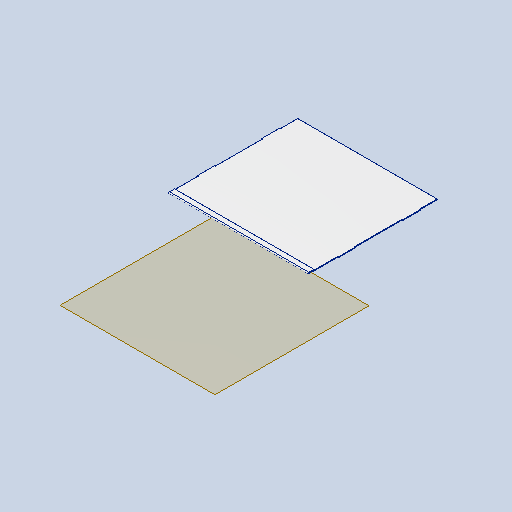
# Autodesk Inventor part: SHELVES
Saved by Autodesk Inventor 2025.2 (Build 292293000, 293)
## iProperties
Created: 2025-03-20
Part Number: SHELVES
Material: Aluminum 6061
Document SubType Name: Sheet Metal
Designer: bless
Density: 2.7 g/cm^3
Sheet Metal Rule: aluminum
Appearance: Aluminum - Flat
Flat Pattern Width: 58.2253 cm
Flat Pattern Length: 60.96 cm
Flat Pattern Area: 3549.42 cm^2
Sheet Metal Width: 22.923 in
Sheet Metal Length: 24.000 in
Sheet Metal Area: 550.161 in^2
Author: bless
Autodesk Inventor part; units mm, degrees
ref_plane "YZ Plane" through (0, 0, 0) normal (1, 0, 0) x (0, 1, 0)
ref_plane "XZ Plane" through (0, 0, 0) normal (0, 1, 0) x (-1, 0, 0)
ref_plane "XY Plane" through (0, 0, 0) normal (0, 0, 1) x (1, 0, 0)
ref_plane "Work Plane1" through (505.636, 20227.0512, -193.0762) normal (0, 1, 0) x (-1, 0, 0)
sketch "Sketch1" plane through (505.636, 20227.0512, -193.0762) normal (0, 1, 0) x (-1, 0, 0)
  circle A0 centre (-63.163, -692.5512) radius 4.7625
  circle A1 centre (-63.163, -444.9012) radius 4.7625
  circle A2 centre (-63.163, -321.0762) radius 4.7625
  circle A3 centre (-63.163, -568.7262) radius 4.7625
  circle A4 centre (-63.163, -816.3762) radius 4.7625
  circle A5 centre (495.637, -321.0762) radius 4.7625
  circle A6 centre (495.637, -444.9012) radius 4.7625
  circle A7 centre (495.637, -568.7262) radius 4.7625
  circle A8 centre (495.637, -692.5512) radius 4.7625
  circle A9 centre (495.637, -816.3762) radius 4.7625
  line L0 (443.2368, -260.7639) -> (-10.7628, -260.7639)
  line L1 (-10.7628, -260.7639) -> (-10.7628, -284.5637)
  line L2 (-10.7628, -284.5637) -> (-17.1128, -284.5637)
  line L3 (-17.1128, -284.5637) -> (-17.1128, -282.9762)
  line L4 (-88.563, -282.9762) -> (-17.1128, -282.9762)
  line L5 (-88.563, -867.1762) -> (-88.563, -282.9762)
  line L6 (521.037, -867.1762) -> (-88.563, -867.1762)
  line L7 (521.037, -282.9762) -> (521.037, -867.1762)
  line L8 (449.5868, -282.9762) -> (521.037, -282.9762)
  line L9 (449.5868, -282.9762) -> (449.5868, -284.5637)
  line L10 (449.5868, -284.5637) -> (443.2368, -284.5637)
  line L11 (443.2368, -284.5637) -> (443.2368, -260.7639)
  line L12 (521.037, -867.1762) -> (-88.563, -867.1762)
  line L13 (-88.563, -867.1762) -> (-88.563, -308.3762)
  line L14 (-88.563, -308.3762) -> (521.037, -308.3762)
  line L15 (521.037, -308.3762) -> (521.037, -867.1762)
  line L16 (-88.563, -790.9762) -> (-85.388, -790.9762)
  line L17 (-85.388, -790.9762) -> (-85.388, -714.7762)
  line L18 (-85.388, -714.7762) -> (-88.563, -714.7762)
  line L19 (-88.563, -714.7762) -> (-88.563, -790.9762)
  line L20 (-85.388, -511.5762) -> (-88.563, -511.5762)
  line L21 (-88.563, -511.5762) -> (-88.563, -435.3762)
  line L22 (-88.563, -435.3762) -> (-85.388, -435.3762)
  line L23 (-85.388, -435.3762) -> (-85.388, -511.5762)
  line L24 (-88.563, -308.3762) -> (-85.388, -308.3762)
  line L25 (-85.388, -308.3762) -> (-85.388, -435.3762)
  line L26 (-85.388, -435.3762) -> (-88.563, -435.3762)
  line L27 (-88.563, -435.3762) -> (-88.563, -308.3762)
  line L28 (-88.563, -511.5762) -> (-85.388, -511.5762)
  line L29 (-85.388, -511.5762) -> (-85.388, -714.7762)
  line L30 (-85.388, -714.7762) -> (-88.563, -714.7762)
  line L31 (-88.563, -714.7762) -> (-88.563, -511.5762)
  line L32 (521.037, -790.9762) -> (517.862, -790.9762)
  line L33 (517.862, -790.9762) -> (517.862, -714.7762)
  line L34 (517.862, -714.7762) -> (521.037, -714.7762)
  line L35 (521.037, -714.7762) -> (521.037, -790.9762)
  line L36 (521.037, -511.5762) -> (517.862, -511.5762)
  line L37 (517.862, -511.5762) -> (517.862, -435.3762)
  line L38 (517.862, -435.3762) -> (521.037, -435.3762)
  line L39 (521.037, -435.3762) -> (521.037, -511.5762)
  line L40 (521.037, -867.1762) -> (517.862, -867.1762)
  line L41 (517.862, -867.1762) -> (517.862, -790.9762)
  line L42 (517.862, -790.9762) -> (521.037, -790.9762)
  line L43 (521.037, -790.9762) -> (521.037, -867.1762)
  line L44 (521.037, -714.7762) -> (517.862, -714.7762)
  line L45 (517.862, -714.7762) -> (517.862, -511.5762)
  line L46 (517.862, -511.5762) -> (521.037, -511.5762)
  line L47 (521.037, -511.5762) -> (521.037, -714.7762)
  line L48 (521.037, -435.3762) -> (517.862, -435.3762)
  line L49 (517.862, -435.3762) -> (517.862, -308.3762)
  line L50 (517.862, -308.3762) -> (521.037, -308.3762)
  line L51 (521.037, -308.3762) -> (521.037, -435.3762)
  line L52 (-88.563, -790.9762) -> (-85.388, -790.9762)
  line L53 (-85.388, -790.9762) -> (-85.388, -867.1762)
  line L54 (-85.388, -867.1762) -> (-88.563, -867.1762)
  line L55 (-88.563, -867.1762) -> (-88.563, -790.9762)
  point P0 (505.636, 193.0762)
  point P1 (521.037, -714.7762)
  point P2 (521.037, -511.5762)
  point P3 (521.037, -435.3762)
  point P4 (-88.563, -435.3762)
  point P5 (-88.563, -511.5762)
  point P6 (-88.563, -714.7762)
  point P7 (-88.563, -790.9762)
  dimension "d0" = 609.6
  dimension "d1" = 558.8
  dimension "d2" = 76.2
  dimension "d3" = 76.2
  dimension "d4" = 3.175
  dimension "d5" = 355.6
  dimension "d6" = 76.2
  dimension "d7" = 3.175
  dimension "d8" = 3.175
  dimension "d9" = 76.2
  dimension "d10" = 76.2
  dimension "d11" = 3.175
  dimension "d12" = 76.2
  dimension "d13" = 355.6
  dimension "d14" = 3.175
  measures "d0" distance of L13.end L14.end
  measures "d1" distance of L12.end L13.end
  measures "d2" distance of L16.end L17.end
  measures "d3" distance between parallel lines of L12 L16
  measures "d4" distance between parallel lines of L19 L17
  measures "d5" distance between parallel lines of L20 L6
  measures "d6" distance of L22.end L20.start
  measures "d7" distance between parallel lines of L13 L23
  measures "d8" distance of L33.end L34.end
  measures "d9" distance of L32.end L33.end
  measures "d10" distance between parallel lines of L6 L32
  measures "d11" distance of L37.end L38.end
  measures "d12" distance of L36.end L37.end
  measures "d13" distance between parallel lines of L6 L36
  measures "d14" distance of L53.end L54.end
extrude "Plate1" add sketch "Sketch1" along normal blind 3.175 contours A0 | A1 | A2 | A3 | A4 | A5 | A6 | A7 | A8 | A9 | L7 L36 L37 L38 | L49 L37 L45 L33 L41 L6 L53 L17 L29 L23 L25 L14 | L22 L23 L20 L5 | L7 L32 L33 L34 | L18 L17 L16 L5
sketch "Sketch2" plane through (-12.2261, 20230.2262, -504.6401) normal (-1, 0, 0) x (0, -1, 0)
  line L0 (3.175, 0) -> (0, 0)
  arc A0 (0, 0) -> (-0.0254, 0) centre (-0.0127, 0) ccw
  line L1 (-0.0254, 0) -> (-0.0254, -22.2123)
  line L2 (-0.0254, -22.2123) -> (-3.2004, -22.2123)
  line L3 (-3.2004, -22.2123) -> (-3.2004, 0)
  arc A1 (3.175, 0) -> (-3.2004, 0) centre (-0.0127, 0) ccw
  constraints: 8 end point, 4 point on circle
hem "Hem1" sketch "Sketch2" thickness 3.175 along (1, 0, 0) edges at (289.3989, 20230.2262, -501.4524)
equation "\"d15\" = Thickness"
equation "\"d16\" = BendReliefWidth"
equation "\"d17\" = BendReliefDepth"
equation "\"d18\" = MinimumRemnant"
equation "\"d19\" = TransitionRadius"
equation "\"d22\" = 0.5 * d21"
equation "\"BendRadius\" = Thickness"
equation "\"BendReliefWidth\" = 2 * Thickness"
equation "\"BendReliefDepth\" = 0.5 * Thickness"
equation "\"CornerReliefSize\" = 4 * Thickness"
equation "\"MinimumRemnant\" = 2 * Thickness"
equation "\"TransitionRadius\" = BendRadius"
equation "\"JacobiRadiusSize\" = BendRadius"
equation "\"GapSize\" = Thickness"
equation "\"Thickness\" = 3.175"
equation "\"d21\" = 0.0254"
body "Solid1"
